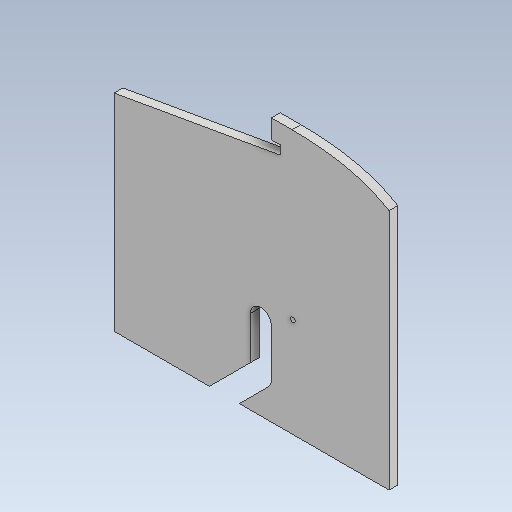
# Autodesk Inventor part: lateral_V2
Saved by Autodesk Inventor 2020 (Build 240168000, 168)
## iProperties
Created: 2020-04-24
Part Number: lateral_V2
Material: Genérico
Document SubType Name: Modeling
Designer: gi-se
Density: 1 g/cm^3
Appearance: Padrão
Author: gi-se
Autodesk Inventor part; units mm, degrees
ref_plane "YZ Plane" through (0, 0, 0) normal (1, 0, 0) x (0, 1, 0)
ref_plane "XZ Plane" through (0, 0, 0) normal (0, 1, 0) x (-1, 0, 0)
ref_plane "XY Plane" through (0, 0, 0) normal (0, 0, 1) x (1, 0, 0)
sketch "Esboço1" plane through (0, 0, 0) normal (0, 0, 1) x (1, 0, 0)
  line L0 (-2.1, 0) -> (-2.1, 1.5) projected
  line L1 (93.5, 0) -> (93.5, 1.5) projected
  line L2 (32.4088, -40) -> (-14.1, -40) projected
  line L3 (0, -40) -> (93.5, -40)
  line L4 (93.5, -40) -> (93.5, 42.2875)
  line L5 (60.5, 49.6356) -> (53.5, 49.6356)
  line L6 (0, 30.2021) -> (0, -40)
  arc A0 (53.5, -11.6) -> (46.3, -11.6) centre (49.9, -11.6) ccw projected
  line L7 (46.3, -11.6) -> (46.3, -26.1088) projected
  line L8 (53.5, -27.6) -> (53.5, -11.6) projected
  arc A1 (52.4456, -30.1456) -> (53.5, -27.6) centre (49.9, -27.6) ccw projected
  line L9 (36.4456, -46.1456) -> (52.4456, -30.1456) projected
  line L10 (46.3, -26.1088) -> (32.4088, -40) projected
  line L11 (65.9, -40) -> (17.9, -40) projected
  circle A2 centre (60.8, -6.2) radius 0.8 projected
  line L12 (-26.1, 0) -> (-26.1, 1.5) projected
  line L13 (-26.1, 25.6) -> (53.5, 39.6356)
  line L14 (53.5, 43.1646) -> (53.5, 49.6356)
  line L15 (53.5, 49.6356) -> (60.5, 49.6356)
  line L16 (110, 1.5) -> (110, 8.5)
  line L17 (60.5, 49.6356) -> (110, 49.6356) construction
  line L18 (110, 49.6356) -> (110, 8.5) construction
  spline S0 degree 2 poles (60.5, 49.6356) (110, 49.6356) (110, 8.5) knots 1 1 1 2 2 2
  line L19 (53.5, 39.6356) -> (56.5, 40.1646)
  line L20 (56.5, 40.1646) -> (56.5, 43.1646)
  line L21 (56.5, 43.1646) -> (53.5, 43.1646)
  point P0 (0, 0)
  point P1 (42.5912, -40)
  dimension "d3" = 10
  dimension "d5" = 7
  dimension "d6" = 7
  dimension "d7" = 3
  constraints: 22 end point, 3 point on line, 3 vertical, 2 parallel, 2 perpendicular, 1 collinear, 1 horizontal, 4 other
  measures "d3" distance of L5.end L13.end
  measures "d5" distance of L5.end L5.start
  measures "d6" distance of L16.start L16.end
  measures "d7" distance of L19.end L20.end
extrude "Extrusão1" add sketch "Esboço1" along normal blind 3 contours L4 L3 L9 A1 L8 A0 L7 L10 L2 L6 L13 L19 L20 L21 L14 L5 S0 L1
